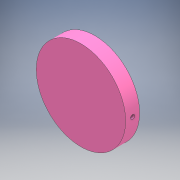
# Autodesk Inventor part: bouchon2
Saved by Autodesk Inventor 2017 (Build 210142000, 142)
## iProperties
Created: 2018-04-06
Part Number: bouchon2
Material: Generic
Document SubType Name: Modeling
Designer: franc
Density: 1 g/cm^3
Appearance: Default
Author: franc
Autodesk Inventor part; units mm, degrees
ref_plane "XZ Plane" through (0, 0, 0) normal (0, 1, 0) x (-1, 0, 0)
ref_plane "XY Plane" through (0, 0, 0) normal (0, 0, 1) x (1, 0, 0)
sketch "Sketch1" plane through (0, 0, 0) normal (0, 1, 0) x (-1, 0, 0)
  circle A0 centre (0, 0) radius 32
  dimension "d0" = 64
  constraints: 1 centre point, 1 coincident
  measures "d0" diameter of A0
extrude "Extrusion1" add sketch "Sketch1" along normal blind 10
sketch "Sketch2" plane through (0, 10, 0) normal (0, 1, 0) x (1, 0, 0)
  circle A0 centre (0, 0) radius 30.5
  dimension "d3" = 61
  constraints: 1 centre point, 1 coincident
  measures "d3" diameter of A0
extrude "Extrusion2" cut sketch "Sketch2" against normal blind 8
ref_plane "Work Plane1" through (32, 0, 0) normal (1, 0, 0) x (0, 1, 0)
sketch "Sketch5" plane through (32, 0, 0) normal (1, 0, 0) x (0, 1, 0)
  circle A0 centre (5, 0) radius 1.5
  line L0 (10, -32) -> (10, 32) projected
  point P0 (0, 0)
  dimension "d7" = 3
  dimension "d8" = 5
  constraints: 1 centre point
  measures "d7" diameter of A0
  measures "d8" distance from line of L0 A0.centre
extrude "Extrusion3" cut sketch "Sketch5" against normal through all
sketch "Esquisse6" plane through (0, 2, 0) normal (0, 1, 0) x (1, 0, 0)
  circle A0 centre (0, 0) radius 25
  dimension "d11" = 50
  constraints: 1 centre point, 1 coincident
  measures "d11" diameter of A0
extrude "Extrusion4" add sketch "Esquisse6" along normal blind 11
body "Solid1"
